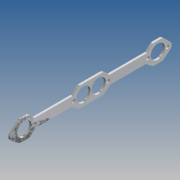
# Autodesk Inventor part: exhaust header plate
Saved by Autodesk Inventor 2013 (Build 170138000, 138)
## iProperties
Created: 2013-02-09
Part Number: exhaust header plate
Material: Steel
Document SubType Name: Sheet Metal
Designer: zhaphod
Density: 1 g/cm^3
Sheet Metal Rule: Default_mm
Author: zhaphod
Autodesk Inventor part; units mm, degrees
ref_plane "YZ Plane" through (0, 0, 0) normal (1, 0, 0) x (0, 1, 0)
ref_plane "XZ Plane" through (0, 0, 0) normal (0, 1, 0) x (-1, 0, 0)
sketch "Sketch1" plane through (0, 0, 0) normal (1, 0, 0) x (0, 1, 0)
  arc A0 (-182.3233, -27.2397) -> (-174.4905, -24.5366) centre (-182.3233, -14.5397) ccw
  line L0 (-156.8537, -10.7176) -> (-174.4905, -24.5366)
  arc A1 (-156.8537, -10.7176) -> (-155.8541, 9.5211) centre (-164.0022, -0.2205) ccw
  line L1 (-174.2578, 27.1272) -> (-155.8541, 9.5211)
  arc A2 (-174.2578, 27.1272) -> (-183.037, 30.6503) centre (-183.037, 17.9503) ccw
  line L2 (-201.4189, 30.6503) -> (-183.037, 30.6503)
  arc A3 (-201.4189, 30.6503) -> (-210.1981, 27.1272) centre (-201.4189, 17.9503) ccw
  line L3 (-223.4861, 14.4151) -> (-210.1981, 27.1272)
  arc A4 (-232.2653, 10.892) -> (-223.4861, 14.4151) centre (-232.2653, 23.592) ccw
  line L4 (-247.1047, 10.892) -> (-232.2653, 10.892)
  line L5 (-247.1047, 10.892) -> (-247.1047, -12.9205)
  line L6 (-229.1736, -12.9205) -> (-247.1047, -12.9205)
  arc A5 (-221.3407, -15.6236) -> (-229.1736, -12.9205) centre (-229.1736, -25.6205) ccw
  line L7 (-209.9654, -24.5366) -> (-221.3407, -15.6236)
  arc A6 (-209.9654, -24.5366) -> (-202.1326, -27.2397) centre (-202.1326, -14.5397) ccw
  line L8 (-182.3233, -27.2397) -> (-202.1326, -27.2397)
  arc A7 (-220.4537, -4.1892) -> (-220.4537, 3.7483) centre (-220.4537, -0.2205) ccw construction
  arc A8 (-220.4537, 3.7483) -> (-220.4537, -4.1892) centre (-220.4537, -0.2205) ccw construction
  arc A9 (-164.0022, -4.1892) -> (-164.0022, 3.7483) centre (-164.0022, -0.2205) ccw construction
  arc A10 (-164.0022, 3.7483) -> (-164.0022, -4.1892) centre (-164.0022, -0.2205) ccw construction
  line L9 (-181.1155, -12.9522) -> (-203.3405, -12.9522)
  arc A11 (-209.6818, -6.2699) -> (-203.3405, -12.9522) centre (-203.3405, -6.6022) ccw
  line L10 (-209.6818, -6.2699) -> (-209.1719, 3.4586)
  arc A12 (-192.228, 19.5378) -> (-209.1719, 3.4586) centre (-192.228, 2.5706) ccw
  arc A13 (-175.284, 3.4586) -> (-192.228, 19.5378) centre (-192.228, 2.5706) ccw
  line L11 (-175.284, 3.4586) -> (-174.7742, -6.2699)
  arc A14 (-181.1155, -12.9522) -> (-174.7742, -6.2699) centre (-181.1155, -6.6022) ccw
  arc A15 (-237.7257, -4.1892) -> (-237.7257, 3.7483) centre (-237.7257, -0.2205) ccw
  arc A16 (-237.7257, 3.7483) -> (-237.7257, -4.1892) centre (-237.7257, -0.2205) ccw
  arc A17 (42.4852, 27.1351) -> (33.7142, 30.6503) centre (33.7142, 17.9503) ccw
  line L12 (-29.131, 30.6503) -> (33.7142, 30.6503)
  arc A18 (-29.131, 30.6503) -> (-37.902, 27.1351) centre (-29.131, 17.9503) ccw
  line L13 (-56.9301, 8.9643) -> (-37.902, 27.1351)
  arc A19 (-56.9301, 8.9643) -> (-55.9818, -10.2253) centre (-48.1592, -0.2205) ccw
  line L14 (-37.6679, -24.5446) -> (-55.9818, -10.2253)
  arc A20 (-37.6679, -24.5446) -> (-29.8453, -27.2397) centre (-29.8453, -14.5397) ccw
  line L15 (34.4285, -27.2397) -> (-29.8453, -27.2397)
  arc A21 (34.4285, -27.2397) -> (42.2511, -24.5446) centre (34.4285, -14.5397) ccw
  line L16 (60.5649, -10.2253) -> (42.2511, -24.5446)
  arc A22 (60.5649, -10.2253) -> (61.5133, 8.9643) centre (52.7423, -0.2205) ccw
  line L17 (42.4852, 27.1351) -> (61.5133, 8.9643)
  arc A23 (-48.1592, 3.7483) -> (-48.1592, -4.1892) centre (-48.1592, -0.2205) ccw construction
  arc A24 (-48.1592, -4.1892) -> (-48.1592, 3.7483) centre (-48.1592, -0.2205) ccw construction
  arc A25 (-2.9895, 3.4586) -> (-19.9334, 19.5378) centre (-19.9334, 2.5706) ccw
  line L18 (-2.4796, -6.2699) -> (-2.9895, 3.4586)
  arc A26 (-8.8209, -12.9522) -> (-2.4796, -6.2699) centre (-8.8209, -6.6022) ccw
  line L19 (-31.0459, -12.9522) -> (-8.8209, -12.9522)
  arc A27 (-37.3872, -6.2699) -> (-31.0459, -12.9522) centre (-31.0459, -6.6022) ccw
  line L20 (-36.8774, 3.4586) -> (-37.3872, -6.2699)
  arc A28 (-19.9334, 19.5378) -> (-36.8774, 3.4586) centre (-19.9334, 2.5706) ccw
  arc A29 (41.4605, 3.4586) -> (24.5166, 19.5378) centre (24.5166, 2.5706) ccw
  line L21 (41.9704, -6.2699) -> (41.4605, 3.4586)
  arc A30 (35.6291, -12.9522) -> (41.9704, -6.2699) centre (35.6291, -6.6022) ccw
  line L22 (13.4041, -12.9522) -> (35.6291, -12.9522)
  arc A31 (7.0628, -6.2699) -> (13.4041, -12.9522) centre (13.4041, -6.6022) ccw
  line L23 (7.5726, 3.4586) -> (7.0628, -6.2699)
  arc A32 (24.5166, 19.5378) -> (7.5726, 3.4586) centre (24.5166, 2.5706) ccw
  arc A33 (52.7423, 3.7483) -> (52.7423, -4.1892) centre (52.7423, -0.2205) ccw construction
  arc A34 (52.7423, -4.1892) -> (52.7423, 3.7483) centre (52.7423, -0.2205) ccw construction
  arc A35 (179.0737, -24.5366) -> (186.9065, -27.2397) centre (186.9065, -14.5397) ccw
  line L24 (206.7158, -27.2397) -> (186.9065, -27.2397)
  arc A36 (206.7158, -27.2397) -> (214.5486, -24.5366) centre (206.7158, -14.5397) ccw
  line L25 (232.1854, -10.7176) -> (214.5486, -24.5366)
  arc A37 (232.1854, -10.7176) -> (233.185, 9.5211) centre (225.0369, -0.2205) ccw
  line L26 (214.7813, 27.1272) -> (233.185, 9.5211)
  arc A38 (214.7813, 27.1272) -> (206.0021, 30.6503) centre (206.0021, 17.9503) ccw
  line L27 (187.6202, 30.6503) -> (206.0021, 30.6503)
  arc A39 (187.6202, 30.6503) -> (178.841, 27.1272) centre (187.6202, 17.9503) ccw
  line L28 (160.4373, 9.5211) -> (178.841, 27.1272)
  arc A40 (160.4373, 9.5211) -> (161.4369, -10.7176) centre (168.5854, -0.2205) ccw
  line L29 (179.0737, -24.5366) -> (161.4369, -10.7176)
  arc A41 (225.0369, 3.7483) -> (225.0369, -4.1892) centre (225.0369, -0.2205) ccw construction
  arc A42 (225.0369, -4.1892) -> (225.0369, 3.7483) centre (225.0369, -0.2205) ccw construction
  arc A43 (213.7551, 3.4586) -> (196.8111, 19.5378) centre (196.8111, 2.5706) ccw
  line L30 (214.2649, -6.2699) -> (213.7551, 3.4586)
  arc A44 (207.9236, -12.9522) -> (214.2649, -6.2699) centre (207.9236, -6.6022) ccw
  line L31 (185.6986, -12.9522) -> (207.9236, -12.9522)
  arc A45 (179.3573, -6.2699) -> (185.6986, -12.9522) centre (185.6986, -6.6022) ccw
  line L32 (179.8672, 3.4586) -> (179.3573, -6.2699)
  arc A46 (196.8111, 19.5378) -> (179.8672, 3.4586) centre (196.8111, 2.5706) ccw
  arc A47 (168.5854, 3.7483) -> (168.5854, -4.1892) centre (168.5854, -0.2205) ccw construction
  arc A48 (168.5854, -4.1892) -> (168.5854, 3.7483) centre (168.5854, -0.2205) ccw construction
  line L33 (224.5369, 4.2795) -> (225.5369, 4.2795)
  line L34 (224.5369, -4.7205) -> (225.5369, -4.7205)
  line L35 (169.0854, 4.2795) -> (168.0854, 4.2795)
  line L36 (168.0854, -4.7205) -> (169.0854, -4.7205)
  line L37 (52.2423, 4.2795) -> (53.2423, 4.2795)
  line L38 (52.2423, -4.7205) -> (53.2423, -4.7205)
  line L39 (-48.6592, 4.2795) -> (-47.6592, 4.2795)
  line L40 (-48.6592, -4.7205) -> (-47.6592, -4.7205)
  line L41 (-164.5022, 4.2795) -> (-163.5022, 4.2795)
  line L42 (-164.5022, -4.7205) -> (-163.5022, -4.7205)
  line L43 (-220.9537, 4.2795) -> (-219.9537, 4.2795)
  line L44 (-220.9537, -4.7205) -> (-219.9537, -4.7205)
  arc A49 (-219.9537, -4.7205) -> (-219.9537, 4.2795) centre (-219.9537, -0.2205) ccw
  arc A50 (-220.9537, 4.2795) -> (-220.9537, -4.7205) centre (-220.9537, -0.2205) ccw
  arc A51 (-163.5022, -4.7205) -> (-163.5022, 4.2795) centre (-163.5022, -0.2205) ccw
  arc A52 (-164.5022, 4.2795) -> (-164.5022, -4.7205) centre (-164.5022, -0.2205) ccw
  arc A53 (-47.6592, -4.7205) -> (-47.6592, 4.2795) centre (-47.6592, -0.2205) ccw
  arc A54 (-48.6592, 4.2795) -> (-48.6592, -4.7205) centre (-48.6592, -0.2205) ccw
  arc A55 (53.2423, -4.7205) -> (53.2423, 4.2795) centre (53.2423, -0.2205) ccw
  arc A56 (52.2423, 4.2795) -> (52.2423, -4.7205) centre (52.2423, -0.2205) ccw
  arc A57 (169.0854, -4.7205) -> (169.0854, 4.2795) centre (169.0854, -0.2205) ccw
  arc A58 (168.0854, 4.2795) -> (168.0854, -4.7205) centre (168.0854, -0.2205) ccw
  arc A59 (225.5369, -4.7205) -> (225.5369, 4.2795) centre (225.5369, -0.2205) ccw
  arc A60 (224.5369, 4.2795) -> (224.5369, -4.7205) centre (224.5369, -0.2205) ccw
  arc A61 (-229.1898, 8.9586) -> (-228.1737, -10.2694) centre (-220.4106, -0.2183) ccw
  line L45 (-223.4861, 14.4151) -> (-229.1898, 8.9586)
  line L46 (-221.3407, -15.6236) -> (-228.2434, -10.2151)
  line L47 (-161.2157, 14.6503) -> (-50.9758, 14.6503)
  line L48 (55.559, 14.6503) -> (165.7989, 14.6503)
  line L49 (162.1033, -11.2397) -> (59.2676, -11.2397)
  line L50 (-54.6844, -11.2397) -> (-157.5201, -11.2397)
  circle A62 centre (-192.228, 2.5706) radius 20.6375
  circle A63 centre (-19.9334, 2.5706) radius 20.6375
  circle A64 centre (24.5166, 2.5706) radius 20.6375
  circle A65 centre (196.8111, 2.5706) radius 20.6375
  point P0 (-220.4537, -4.7205)
  point P1 (-164.0022, -4.7205)
  point P2 (-48.1592, -4.7205)
  point P3 (52.7423, -4.7205)
  point P4 (168.5854, -4.7205)
  point P5 (225.0369, -4.7205)
  dimension "d9" = 1
  dimension "d11" = 4.5
  dimension "d12" = 1
  dimension "d13" = 1
  dimension "d14" = 1
  dimension "d15" = 1
  dimension "d16" = 1
  dimension "d19" = 16
  dimension "d20" = 16
  dimension "d22" = 41.275
  measures "d9" distance of L43.start L43.end
  measures "d11" radius of A50
  measures "d12" distance of L41.start L41.end
  measures "d13" distance of L39.start L39.end
  measures "d14" distance of L37.start L37.end
  measures "d15" distance of L35.start L35.end
  measures "d16" distance of L33.start L33.end
  measures "d19" distance between parallel lines of L12 L47
  measures "d20" distance between parallel lines of L50 L15
  measures "d22" diameter of A62
extrude "Plate1" add sketch "Sketch1" along normal blind 6 contours L8 A6 L7 L46 A61 L45 L3 A3 L2 A2 L1 A1 L0 A0 | L0 A1 L1 L47 L13 A19 L14 L50 | L14 A19 L13 A18 L12 A17 L17 A22 L16 A21 L15 A20 | L16 A22 L17 L48 L28 A40 L29 L49 | L29 A40 L28 A39 L27 A38 L26 A37 L25 A36 L24 A35
ref_plane "Work Plane1" through (0, -19.9334, 2.5706) normal (0, 0, 1) x (1, 0, 0)
equation "\"d12\" = d9"
equation "\"d13\" = d9"
equation "\"d14\" = d9"
equation "\"d15\" = d9"
equation "\"d16\" = d9"
equation "\"BendRadius\" = Thickness"
equation "\"BendReliefWidth\" = Thickness"
equation "\"BendReliefDepth\" = 0.5 * Thickness"
equation "\"CornerReliefSize\" = 4 * Thickness"
equation "\"MinimumRemnant\" = 2 * Thickness"
equation "\"TransitionRadius\" = BendRadius"
equation "\"JacobiRadiusSize\" = BendRadius"
equation "\"GapSize\" = Thickness"
equation "\"d18\" = d17"
equation "\"d21\" = BendRadius"
equation "\"Thickness\" = 6"
equation "\"d17\" = 8"
body "Solid1"
